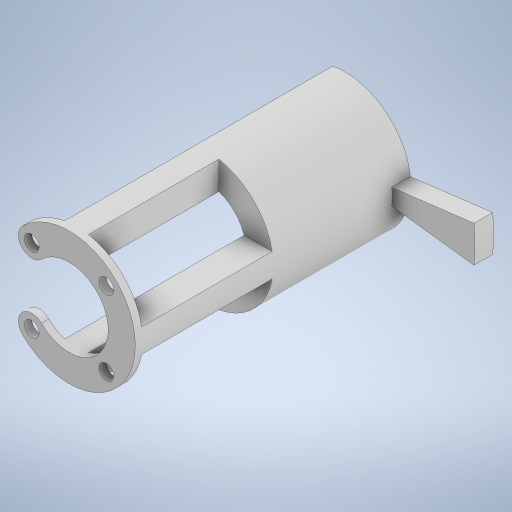
# Autodesk Inventor part: stop_rotador_1
Saved by Autodesk Inventor 2024 (Build 280153000, 153)
## iProperties
Created: 2023-03-25
Part Number: stop_rotador_1
Material: Generic
Document SubType Name: Modeling
Designer: ferna
Density: 1 g/cm^3
Appearance: Default
Author: ferna
Autodesk Inventor part; units mm, degrees
ref_plane "YZ Plane" through (0, 0, 0) normal (1, 0, 0) x (0, 1, 0)
ref_plane "XZ Plane" through (0, 0, 0) normal (0, 1, 0) x (-1, 0, 0)
ref_plane "XY Plane" through (0, 0, 0) normal (0, 0, 1) x (1, 0, 0)
sketch "Sketch1" plane through (0, 0, 0) normal (0, 0, 1) x (1, 0, 0)
  circle A0 centre (0, 0) radius 10
  circle A1 centre (0, 0) radius 18.4566
  circle A2 centre (10, -10) radius 2
  circle A3 centre (10, 10) radius 2
  circle A4 centre (-10, 10) radius 2
  circle A5 centre (-10, -10) radius 2
  circle A6 centre (-10, -10) radius 2
  circle A7 centre (-10, -10) radius 4.1421
  circle A8 centre (0, 0) radius 10
  circle A9 centre (-10, 10) radius 2
  circle A10 centre (-10, 10) radius 4.1421
  circle A11 centre (0, 0) radius 10.5
  circle A12 centre (-10, -10) radius 3.6421
  circle A13 centre (-10, 10) radius 3.6421
  line L0 (-7.4246, 7.4246) -> (-10, 10)
  line L1 (-10, 10) -> (-11.4142, 11.4142)
  line L2 (-11.4142, 11.4142) -> (-12.5754, 12.5754)
  circle A14 centre (0, 0) radius 17.7843
  point P0 (-7.4246, -7.4246)
  point P1 (-12.5754, -12.5754)
  dimension "d0" = 21
  constraints: 12 centre point, 6 coincident, 6 end point, 2 point on circle, 2 tangent, 1 point on line, 11 other
extrude "Extrusion1" add sketch "Sketch1" along normal blind 2 contours A11 A13 A14 A10 | A10 A14 A7 A11 | A7 A14 A12 A11 | L0 A4 L2 A13 | A13 L2 A4 L0 | A12 picked at (-6.0591, 10.307) picked at (12.8553, 5.0845) picked at (-6.0591, -10.307)
sketch "Sketch2" plane through (0, 0, 0) normal (0, 0, -1) x (-1, 0, 0)
  arc A0 (12.5754, -12.5754) -> (7.4246, -7.4246) centre (10, -10) ccw projected
  arc A1 (7.4246, 7.4246) -> (7.4246, -7.4246) centre (0, 0) ccw projected
  arc A2 (7.4246, 7.4246) -> (12.5754, 12.5754) centre (10, 10) ccw projected
  arc A3 (12.5754, 12.5754) -> (12.5754, -12.5754) centre (0, 0) ccw projected
  circle A4 centre (10, 10) radius 2 projected
  circle A5 centre (10, -10) radius 2 projected
  circle A6 centre (-10, -10) radius 2 projected
  circle A7 centre (-10, 10) radius 2 projected
  arc A8 (7.4246, 7.4246) -> (7.4246, -7.4246) centre (0, 0) ccw projected
  line L0 (-10, 3.2016) -> (-17.4937, 3.2016)
  arc A9 (12.5754, 12.5754) -> (12.5754, -12.5754) centre (0, 0) ccw projected
  line L1 (-10, -3.2016) -> (-17.4937, -3.2016)
  line L2 (-3.2016, -10) -> (-3.2016, -17.4937)
  line L3 (3.2016, -10) -> (3.2016, -17.4937)
  line L4 (3.2016, 10) -> (3.2016, 17.4937)
  line L5 (-3.2016, 17.4937) -> (-3.2016, 10)
  constraints: 12 end point, 12 point on circle, 4 point on line, 2 parallel, 1 horizontal, 1 perpendicular
extrude "Extrusion2" add sketch "Sketch2" along normal blind 10 contours A3 L2 A1 L3 | A3 L0 A1 L1 | A3 L4 A1 L5
sketch "Sketch4" plane through (0, 0, -10) normal (0, 0, -1) x (-1, 0, 0)
  arc A0 (3.2016, 10) -> (-3.2016, 10) centre (0, 0) ccw projected
  line L0 (3.2016, 10) -> (3.2016, 17.4937) projected
  arc A1 (3.2016, 17.4937) -> (-3.2016, 17.4937) centre (0, 0) ccw projected
  line L1 (-3.2016, 17.4937) -> (-3.2016, 10) projected
  arc A2 (-3.2016, -10) -> (3.2016, -10) centre (0, 0) ccw projected
  line L2 (-3.2016, -10) -> (-3.2016, -17.4937) projected
  arc A3 (-3.2016, -17.4937) -> (3.2016, -17.4937) centre (0, 0) ccw projected
  line L3 (3.2016, -17.4937) -> (3.2016, -10) projected
  circle A4 centre (-10, -10) radius 2 projected
  line L4 (-3.2016, -17.4937) -> (-3.2016, -10) projected
  arc A5 (-10, -3.2016) -> (-3.2016, -10) centre (0, 0) ccw projected
  line L5 (-10, -3.2016) -> (-17.4937, -3.2016) projected
  arc A6 (-17.4937, -3.2016) -> (-3.2016, -17.4937) centre (0, 0) ccw projected
  arc A7 (-10, 3.2016) -> (-10, -3.2016) centre (0, 0) ccw projected
  line L6 (-10, 3.2016) -> (-17.4937, 3.2016) projected
  arc A8 (-17.4937, 3.2016) -> (-17.4937, -3.2016) centre (0, 0) ccw projected
  line L7 (-17.4937, -3.2016) -> (-10, -3.2016) projected
  line L8 (-17.4937, 3.2016) -> (-10, 3.2016) projected
  arc A9 (-3.2016, 10) -> (-10, 3.2016) centre (0, 0) ccw projected
  line L9 (-3.2016, 10) -> (-3.2016, 17.4937) projected
  arc A10 (-3.2016, 17.4937) -> (-17.4937, 3.2016) centre (0, 0) ccw projected
  circle A11 centre (-10, 10) radius 2 projected
extrude "Extrusion3" add sketch "Sketch4" along normal blind 62 contours A0 L1 A1 L0 | A9 L6 A10 L1 | A7 L5 A8 L6 | A5 L2 A6 L5 | A2 L3 A3 L2 | A4 | A11
sketch "Sketch5" plane through (0, 0, -72) normal (0, 0, -1) x (-1, 0, 0)
  line L0 (0, 0) -> (-40, 0)
  arc A0 (-40, 0) -> (-39.7018, -4.8748) centre (0, 0) ccw
  line L1 (0, 0) -> (-39.7018, -4.8748) construction
  line L2 (0, 0) -> (-40, 0) construction
  arc A1 (-39.7018, 4.8748) -> (-40, 0) centre (0, 0) ccw
  line L3 (-39.7018, 4.8748) -> (0, 0)
  line L4 (0, 0) -> (-39.7018, -4.8748)
  arc A2 (3.2016, 17.4937) -> (3.2016, -17.4937) centre (0, 0) ccw projected
  point P0 (-17.6517, -2.1674)
  point P1 (-17.6517, 2.1674)
  dimension "d7" = 40
  dimension "d8" = 7
  constraints: 10 end point, 5 point on circle, 2 centre point, 2 coincident, 1 collinear, 1 concentric, 1 horizontal
  measures "d7" distance of L0.start L0.end
  measures "d8" angle of L2 L1
extrude "Extrusion4" add sketch "Sketch5" against normal blind 5 contours A2 L4 A0 L0 | L0 A1 L3 A2
sketch "Sketch6" plane through (0, 0, -10) normal (0, 0, 1) x (1, 0, 0)
  line L0 (10, 3.2016) -> (17.4937, 3.2016) projected
  arc A0 (17.4937, 3.2016) -> (3.2016, 17.4937) centre (0, 0) ccw projected
  line L1 (3.2016, 17.4937) -> (3.2016, 10) projected
  arc A1 (10, 3.2016) -> (3.2016, 10) centre (0, 0) ccw projected
  line L2 (3.2016, -10) -> (3.2016, -17.4937) projected
  arc A2 (3.2016, -17.4937) -> (17.4937, -3.2016) centre (0, 0) ccw projected
  line L3 (17.4937, -3.2016) -> (10, -3.2016) projected
  arc A3 (3.2016, -10) -> (10, -3.2016) centre (0, 0) ccw projected
extrude "Extrusion5" cut sketch "Sketch6" against normal blind 25
body "Solid1"
